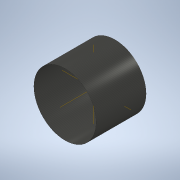
# Autodesk Inventor part: BasicBuoy
Saved by Autodesk Inventor 2020 (Build 240168000, 168)
## iProperties
Created: 2020-06-15
Part Number: BasicBuoy
Material: Steel
Document SubType Name: Modeling
Designer: Freeman
Mass: 7.66171e+07 g
Surface Area: 6.57675e+06 cm^2
Volume: 9.76014e+06 cm^3
Density: 7.85 g/cm^3
Appearance: Plate
Author: Freeman
Autodesk Inventor part; units mm, degrees
ref_plane "YZ Plane" through (0, 0, 0) normal (1, 0, 0) x (0, 1, 0)
ref_plane "XZ Plane" through (0, 0, 0) normal (0, 1, 0) x (-1, 0, 0)
ref_plane "XY Plane" through (0, 0, 0) normal (0, 0, 1) x (1, 0, 0)
sketch "Sketch2" plane through (0, 0, 0) normal (1, 0, 0) x (0, 1, 0)
  line L0 (0, -3081.26) -> (0, -3491.26)
  line L1 (0, -3491.26) -> (5000, -3491.26)
  line L2 (5000, -3491.26) -> (5000, 4508.74)
  line L3 (5000, 4508.74) -> (4966, 4508.74)
  line L4 (4966, 4508.74) -> (4966, -3475.26)
  line L5 (4966, -3475.26) -> (60, -3475.26)
  line L6 (60, -3475.26) -> (60, -3081.26)
  line L7 (60, -3081.26) -> (0, -3081.26)
  line L8 (0, -5091.26) -> (0, 6108.74) projected
  line L9 (-1000, 0) -> (6000, 0) projected
  point P0 (0, 0)
  dimension "d0" = 8000
  dimension "d1" = 410
  dimension "d2" = 7984
  dimension "d3" = 60
  dimension "d4" = 34
  dimension "d5" = 16
  dimension "d6" = 5000
  dimension "d7" = 0
  dimension "d10" = 3475.26
  constraints: 16 end point, 7 perpendicular, 1 vertical
  measures "d0" distance of L1.end L2.end
  measures "d1" distance of L0.start L0.end
  measures "d2" distance of L3.end L4.end
  measures "d3" distance of L6.end L0.start
  measures "d4" distance of L2.end L3.end
  measures "d5" distance between parallel lines of L1 L5
  measures "d6" distance of L0.end L1.end
  measures "d7" distance between parallel lines of L8 L0
  measures "d10" distance between parallel lines of L5 L9
revolve "Revolution1" add sketch "Sketch2" angle 360 about axis through (0, 0, -10) along (0, 0, 1) contours L7 L6 L5 L4 L9 L2 L1 L0 | L4 L3 L2 L9
body "Solid1"
